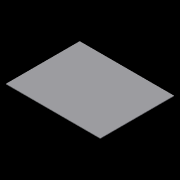
# Autodesk Inventor part: 3d_JacintoDevKit_Addon - Jacinto
Saved by Autodesk Inventor 2018.3 (Build 223284000, 284)
## iProperties
Created: 2026-02-26
Part Number: 3d_JacintoDevKit_Addon - Jacinto
Material: Genérico
Document SubType Name: Modeling
Designer: aca6
Density: 1 g/cm^3
Appearance: Valor por defecto
Author: aca6
Autodesk Inventor part; units mm, degrees
ref_plane "YZ Plane" through (0, 0, 0) normal (1, 0, 0) x (0, 1, 0)
ref_plane "XZ Plane" through (0, 0, 0) normal (0, 1, 0) x (-1, 0, 0)
ref_plane "XY Plane" through (0, 0, 0) normal (0, 0, 1) x (1, 0, 0)
sketch "Sketch1" plane through (0, 0, 0) normal (0, 0, 1) x (1, 0, 0)
  line L0 (-121.88, 95.25) -> (121.88, 95.25)
  line L1 (121.88, 95.25) -> (121.88, -95.25)
  line L2 (121.88, -95.25) -> (-121.88, -95.25)
  line L3 (-121.88, -95.25) -> (-121.88, 95.25)
  line L4 (0, 0) -> (0, 94.2706) construction
  line L5 (0, 0) -> (62.82, 0) construction
  dimension "d0" = 243.76
  dimension "d1" = 190.5
  constraints: 12 end point, 3 horizontal, 2 parallel, 2 vertical, 1 perpendicular, 2 other
  measures "d0" distance between parallel lines of L1 L3
  measures "d1" distance of L0.end L1.end
extrude "Extrusion1" add sketch "Sketch1" along normal blind 1.6
body "Solid1"
